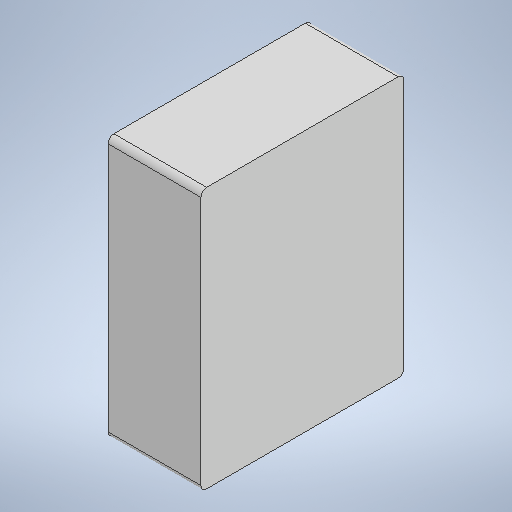
# Autodesk Inventor part: Base
Saved by Autodesk Inventor 2025 (Build 290162000, 162)
## iProperties
Created: 2024-05-29
Part Number: Base
Material: Générique
Document SubType Name: Modeling
Designer: luc4s
Density: 1 g/cm^3
Appearance: Par défaut
Author: luc4s
Autodesk Inventor part; units mm, degrees
ref_plane "YZ Plane" through (0, 0, 0) normal (1, 0, 0) x (0, 1, 0)
ref_plane "XZ Plane" through (0, 0, 0) normal (0, 1, 0) x (-1, 0, 0)
ref_plane "XY Plane" through (0, 0, 0) normal (0, 0, 1) x (1, 0, 0)
sketch "Esquisse1" plane through (0, 0, 0) normal (1, 0, 0) x (0, 1, 0)
  line L0 (45, 35) -> (-45, 35)
  line L1 (-45, 35) -> (-45, -35)
  line L2 (-45, -35) -> (45, -35)
  line L3 (45, -35) -> (45, 35)
  line L4 (0, 39.01) -> (0, -54.7883) construction
  line L5 (27.6574, 0) -> (-32.6664, 0) construction
  point P0 (0, 0)
  dimension "d0" = 70
  dimension "d1" = 90
  constraints: 12 end point, 2 horizontal, 2 parallel, 2 point on line, 1 perpendicular, 1 vertical, 2 other
  measures "d0" distance of L2.end L0.start
  measures "d1" distance of L1.end L2.end
extrude "Extrusion1" add sketch "Esquisse1" along normal blind 2
sketch "Esquisse2" plane through (0, 0, 0) normal (-1, 0, 0) x (0, 0, 1)
  line L0 (35, -45) -> (-35, -45) projected
  line L1 (-35, 45) -> (35, 45) projected
  line L2 (-35, -45) -> (35, -45)
  line L3 (35, -45) -> (35, 45)
  line L4 (35, 45) -> (-35, 45)
  line L5 (-35, 45) -> (-35, -45)
  line L6 (-33, -43) -> (33, -43)
  line L7 (33, -43) -> (33, 43)
  line L8 (33, 43) -> (-33, 43)
  line L9 (-33, 43) -> (-33, -43)
  point P0 (0, 0)
  dimension "d4" = 2
  dimension "d5" = 2
  dimension "d6" = 2
  dimension "d7" = 2
  constraints: 16 end point, 4 parallel, 2 horizontal, 2 perpendicular
  measures "d4" distance from line of L0 L6.start
  measures "d5" distance from line of L5 L6.start
  measures "d6" distance from line of L3 L7.end
  measures "d7" distance from line of L1 L7.end
extrude "Extrusion2" add sketch "Esquisse2" along normal blind 30
fillet "Congé1" radius 2 2 edges at (-14, 45, 35) (-14, -45, 35)
fillet "Congé2" radius 2 2 edges at (-14, 45, -35) (-14, -45, -35)
